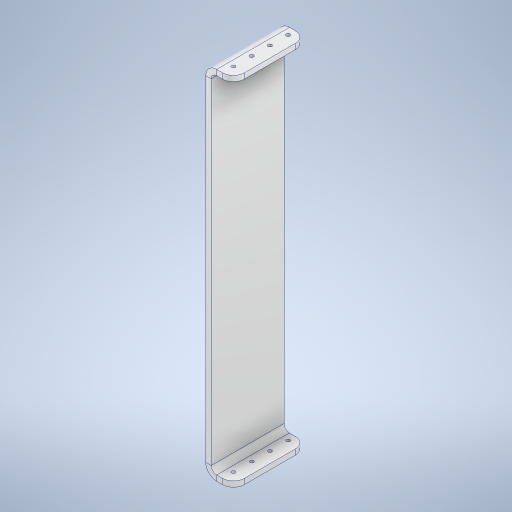
# Autodesk Inventor part: ramp
Saved by Autodesk Inventor 2023 (Build 270158000, 158)
## iProperties
Created: 2022-05-09
Part Number: ramp
Material: Aluminum 6061
Document SubType Name: Sheet Metal
Designer: Dan
Density: 2.7 g/cm^3
Sheet Metal Rule: Default_mm
Appearance: Aluminum - Flat
Mass: 207.914 g
Surface Area: 535.297 cm^2
Volume: 77.0053 cm^3
BendRadius: 3.000 mm
BendReliefWidth: 3.000 mm
BendReliefDepth: 1.500 mm
CornerReliefSize: 12.000 mm
MinimumRemnant: 6.000 mm
TransitionRadius: 3.000 mm
JacobiRadiusSize: 3.000 mm
GapSize: 3.000 mm
Author: Dan
Autodesk Inventor part; units mm, degrees
ref_plane "YZ Plane" through (0, 0, 0) normal (1, 0, 0) x (0, 1, 0)
ref_plane "XZ Plane" through (0, 0, 0) normal (0, 1, 0) x (-1, 0, 0)
ref_plane "XY Plane" through (0, 0, 0) normal (0, 0, 1) x (1, 0, 0)
sketch "Sketch1" plane through (0, 0, 0) normal (0, 1, 0) x (-1, 0, 0)
  line L0 (0, 0) -> (-108, 0)
  line L1 (-108, -40) -> (0, -40)
  line L2 (0, 0) -> (0, -40)
  circle A0 centre (-102, -36) radius 1
  line L3 (-92, -40) -> (-92, 0)
  line L4 (-102, -40) -> (-102, 0) construction
  circle A1 centre (-102, -26) radius 1
  circle A2 centre (-102, -16) radius 1
  circle A3 centre (-102, -6) radius 1
  line L5 (-102, -36) -> (-102, -26)
  line L6 (-92, -40) -> (0, -40)
  line L7 (0, -40) -> (0, -50)
  line L8 (0, -50) -> (-92, -50)
  line L9 (-92, -50) -> (-92, -40)
  line L10 (-108, -40) -> (-108, 0)
  dimension "d50" = 2
  dimension "d84" = 10
  dimension "d87" = 10
  dimension "d92" = 6
  dimension "d96" = 92
  dimension "d97" = 40
  dimension "d132" = 10
  dimension "d151" = 6
  dimension "d152" = 90
  constraints: 23 end point, 5 parallel, 4 centre point, 4 point on line, 2 coincident, 2 horizontal, 2 vertical, 1 perpendicular, 6 other
  measures "d50" diameter of A0
  measures "d84" distance between parallel lines of L3 L4
  measures "d87" distance of L5.start L5.end
  measures "d92" distance from line of L0 A3.centre
  measures "d96" distance of L3.start L1.end
  measures "d97" distance of L0.start L1.end
  measures "d132" distance of L3.start L8.end
  measures "d151" distance between parallel lines of L10 L4
  measures "d152" angle of L6 L3
extrude "Plate1" add sketch "Sketch1" along normal blind 3 contours L2 L1 L3 L0 | L3 L1 L10 L0
fold "Fold2" angle 90 bend radius 3 thickness 3 k factor 0.44 line from (92, 0, -40) to (92, 0, 0) line at bend end moving side (-1, 0, 0) folds toward (0, -1, 0)
fillet "Corner Round2" radius 6 2 edges at (108, 1.5, -40) (108, 1.5, 0)
mirror "Mirror2" about plane through (95.7858, -95, 0) normal (0, -1, 0)
equation "\"d2\" = Thickness"
equation "\"d98\" = BendReliefWidth"
equation "\"d99\" = BendReliefDepth"
equation "\"d100\" = MinimumRemnant"
equation "\"d101\" = TransitionRadius"
equation "\"d103\" = BendRadius"
equation "\"BendRadius\" = Thickness"
equation "\"BendReliefWidth\" = Thickness"
equation "\"BendReliefDepth\" = 0.5 * Thickness"
equation "\"CornerReliefSize\" = 4 * Thickness"
equation "\"MinimumRemnant\" = 2 * Thickness"
equation "\"TransitionRadius\" = BendRadius"
equation "\"JacobiRadiusSize\" = BendRadius"
equation "\"GapSize\" = Thickness"
equation "\"Thickness\" = 3"
body "Solid1"
